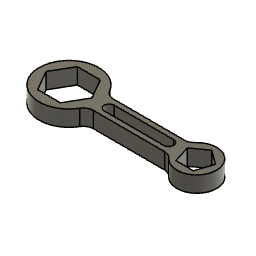
EX2 (Autodesk Fusion 360 design; units mm, degrees)
Autodesk Fusion 360 part; units mm, degrees
sketch "Sketch1" plane through (0, 0, 0) normal (0, 1, 0) x (1, 0, 0)
  line L0 (-11.547, 20) -> (-23.094, 0)
  line L1 (-23.094, 0) -> (-11.547, -20)
  line L2 (-11.547, -20) -> (11.547, -20)
  line L3 (11.547, -20) -> (23.094, 0)
  line L4 (23.094, 0) -> (11.547, 20)
  line L5 (11.547, 20) -> (-11.547, 20)
  line L6 (129.0614, 14.7865) -> (114.7531, 4.4803)
  line L7 (114.7531, 4.4803) -> (120.1333, -12.3124)
  line L8 (120.1333, -12.3124) -> (137.7667, -12.3847)
  line L9 (137.7667, -12.3847) -> (143.2846, 4.3633)
  line L10 (143.2846, 4.3633) -> (129.0614, 14.7865)
  line L11 (34.6575, 9.9427) -> (106.6557, 9.8236)
  line L12 (34.6244, -10.0573) -> (106.6226, -10.1764)
  arc A0 (26.0055, 14.957) -> (34.6575, 9.9427) centre (34.6741, 19.9427) ccw
  arc A1 (34.6244, -10.0573) -> (25.9559, -15.043) centre (34.6079, -20.0573) ccw
  arc A2 (114.0707, -13.5221) -> (106.6226, -10.1764) centre (106.6061, -20.1764) ccw
  arc A3 (106.6557, 9.8236) -> (114.1148, 13.1446) centre (106.6723, 19.8235) ccw
  circle A4 centre (0, 0) radius 30
  circle A5 centre (128.9998, -0.2134) radius 20
  line L13 (100.6483, 4.8335) -> (40.6484, 4.9328)
  arc A6 (40.6484, 4.9328) -> (40.6318, -5.0672) centre (40.6401, -0.0672) ccw
  line L14 (40.6318, -5.0672) -> (100.6318, -5.1665)
  arc A7 (100.6318, -5.1665) -> (100.6483, 4.8335) centre (100.64, -0.1665) ccw
  point P0 (128.9998, -0.2134)
  dimension "d1" = 60
  dimension "d5" = 40
  dimension "d6" = 15
  dimension "d7" = 129
  dimension "d8" = 20
  dimension "d13" = 10
  dimension "d20" = 10
  dimension "d22" = 20
  constraint coincident A4.centre origin
  constraint tangent L11 A0
  constraint tangent A0 A4
  constraint tangent L12 A1
  constraint tangent A1 A4
  constraint equal A0 A1
  constraint tangent A2 A5
  constraint tangent L12 A2
  constraint equal A0 A2
  constraint tangent L11 A3
  constraint tangent A3 A5
  constraint equal A0 A3
  constraint coincident A1.end A4
  constraint coincident A2.start A5
  constraint tangent L13 A6
  constraint tangent A6 L14
  constraint parallel L13 L14
  constraint tangent L14 A7
  constraint tangent L13 A7
  measures "d1" diameter of A4
  measures "d5" diameter of A5
  measures "d6" distance of L6.start P0
  measures "d7" distance of A4.centre P0
  measures "d8" distance of A4.centre L2
  measures "d13" radius of A0
  measures "d20" distance of L13 L14
  measures "d22" distance of L11 L12
extrude "Extrude1" add sketch "Sketch1" along normal blind 8 and the other way blind 8
